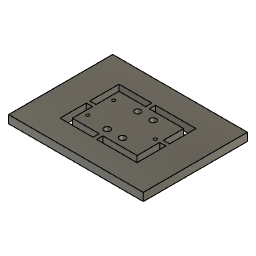
Usinage v5 (Autodesk Fusion 360 design; units mm, degrees)
Autodesk Fusion 360 part; units mm, degrees
sketch "Esquisse1" plane through (0, 0, 0) normal (0, 0, 1) x (1, 0, 0)
  line L0 (-35, 50) -> (75, 50)
  line L1 (75, 50) -> (75, -35)
  line L2 (75, -35) -> (-35, -35)
  line L3 (-35, -35) -> (-35, 50)
  circle A0 centre (28.055, -5) radius 2.5
  circle A1 centre (-2.15, 18) radius 1.25
  circle A2 centre (15.555, -5) radius 2.5
  circle A3 centre (-2.15, -3) radius 1.25
  circle A4 centre (15.555, 20) radius 2.5
  circle A5 centre (42.25, 7.5) radius 1.25
  circle A6 centre (28.055, 20) radius 2.5
  line L4 (-11.4, 4.8329) -> (-6.4, 4.8329)
  line L5 (-11.4, 7.8329) -> (-6.4, 7.8329)
  line L6 (15.3682, 31.55) -> (15.3682, 26.55)
  line L7 (18.3682, 31.55) -> (18.3682, 26.55)
  line L8 (46.4, 10) -> (51.4, 10)
  line L9 (46.4, 7) -> (51.4, 7)
  line L10 (15.555, -11.55) -> (15.555, -16.55)
  line L11 (18.555, -11.55) -> (18.555, -16.55)
  line L12 (-11.4, 31.55) -> (15.3682, 31.55)
  line L13 (18.3682, 31.55) -> (51.4, 31.55)
  line L14 (46.4, 26.55) -> (18.3682, 26.55)
  line L15 (15.3682, 26.55) -> (-6.4, 26.55)
  line L16 (51.4, 31.55) -> (51.4, 10)
  line L17 (51.4, 7) -> (51.4, -16.55)
  line L18 (46.4, -11.55) -> (46.4, 7)
  line L19 (46.4, 10) -> (46.4, 26.55)
  line L20 (-6.4, -11.55) -> (15.555, -11.55)
  line L21 (18.555, -11.55) -> (46.4, -11.55)
  line L22 (51.4, -16.55) -> (18.555, -16.55)
  line L23 (15.555, -16.55) -> (-11.4, -16.55)
  line L24 (-11.4, -16.55) -> (-11.4, 4.8329)
  line L25 (-11.4, 7.8329) -> (-11.4, 31.55)
  line L26 (-6.4, 26.55) -> (-6.4, 7.8329)
  line L27 (-6.4, 4.8329) -> (-6.4, -11.55)
  point P0 (20, 10)
  dimension "d1" = 110
  dimension "d2" = 85
  dimension "d3" = 2.5
  dimension "d4" = 2.5
  dimension "d5" = 5
  dimension "d6" = 5
  dimension "d7" = 5
  dimension "d8" = 5
  dimension "d9" = 2.5
  dimension "d10" = 38.1
  dimension "d11" = 52.8
  dimension "d12" = 6.55
  dimension "d13" = 6.55
  dimension "d14" = 8.55
  dimension "d15" = 8.55
  dimension "d16" = 6.55
  dimension "d17" = 6.55
  dimension "d18" = 19.05
  dimension "d19" = 4.15
  dimension "d20" = 18.345
  dimension "d21" = 30.845
  dimension "d22" = 4.25
  dimension "d23" = 4.25
  dimension "d24" = 21.955
  dimension "d25" = 18.345
  dimension "d26" = 23.45
  dimension "d27" = 38.1
  dimension "d28" = 52.8
  dimension "d30" = 28.6
  dimension "d35" = 5
  dimension "d36" = 5
  dimension "d37" = 5
  dimension "d38" = 5
  dimension "d39" = 3
  dimension "d40" = 3
  dimension "d41" = 3
  dimension "d42" = 3
  constraint horizontal L0
  constraint vertical L1
  constraint horizontal L2
  constraint vertical L3
  constraint parallel L3 L26
  constraint horizontal L12
  constraint vertical L16
  constraint horizontal L22
  constraint vertical L24
  constraint coincident L4.end L26
  constraint perpendicular L4 L26
  constraint coincident L5.start L24
  constraint perpendicular L5 L26
  constraint coincident L6.end L14
  constraint perpendicular L6 L14
  constraint coincident L7.start L12
  constraint perpendicular L7 L14
  constraint coincident L8.start L18
  constraint perpendicular L8 L16
  constraint coincident L9.end L16
  constraint perpendicular L9 L16
  constraint coincident L10.end L22
  constraint perpendicular L10 L22
  constraint coincident L11.start L20
  constraint perpendicular L11 L22
  constraint collinear L12 L13
  constraint collinear L14 L15
  constraint collinear L16 L17
  constraint collinear L18 L19
  constraint collinear L20 L21
  constraint collinear L22 L23
  constraint collinear L24 L25
  constraint collinear L26 L27
  measures "d1" distance of L1 L3
  measures "d2" distance of L0 L2
  measures "d3" diameter of A1
  measures "d4" diameter of A3
  measures "d5" diameter of A4
  measures "d6" diameter of A6
  measures "d7" diameter of A2
  measures "d8" diameter of A0
  measures "d9" diameter of A5
  measures "d10" distance of L15.end L20.start
  measures "d11" distance of L15.end L14.start
  measures "d12" distance of A6.centre L14
  measures "d13" distance of A4.centre L14
  measures "d14" distance of A1.centre L14
  measures "d15" distance of A3.centre L20
  measures "d16" distance of A2.centre L20
  measures "d17" distance of A0.centre L20
  measures "d18" distance of A5.centre L20
  measures "d19" distance of A5.centre L18
  measures "d20" distance of A6.centre L18
  measures "d21" distance of A4.centre L18
  measures "d22" distance of A1.centre L26
  measures "d23" distance of A3.centre L26
  measures "d24" distance of A2.centre L26
  measures "d25" distance of A0.centre L18
  measures "d26" distance of L0 L14
  measures "d27" distance of L18.start L14.start
  measures "d28" distance of L20.start L18.start
  measures "d30" distance of L3 L26
  measures "d35" distance of L24 L26
  measures "d36" distance of L12 L14
  measures "d37" distance of L20 L22
  measures "d38" distance of L16 L18
  measures "d39" distance of L4 L5
  measures "d40" distance of L10 L11
  measures "d41" distance of L8 L9
  measures "d42" distance of L6 L7
extrude "Extrusion3" add sketch "Esquisse1" along normal blind 6.5 contours L0 L1 L2 L3 | A1 | A3 | A5
sketch "Esquisse3" plane through (0, 0, 6.5) normal (0, 0, 1) x (-1, 0, 0)
  circle A0 centre (-15.555, -20) radius 2.5
  circle A1 centre (-28.055, -20) radius 2.5
  line L0 (11.4, -4.8329) -> (6.4, -4.8329)
  line L1 (6.4, -4.8329) -> (6.4, 11.55)
  line L2 (6.4, 11.55) -> (-15.555, 11.55)
  line L3 (-15.555, 11.55) -> (-15.555, 16.55)
  line L4 (-15.555, 16.55) -> (11.4, 16.55)
  line L5 (11.4, 16.55) -> (11.4, -4.8329)
  line L6 (-18.3682, -26.55) -> (-18.3682, -31.55)
  line L7 (-18.3682, -31.55) -> (-51.4, -31.55)
  line L8 (-51.4, -31.55) -> (-51.4, -10)
  line L9 (-51.4, -10) -> (-46.4, -10)
  line L10 (-46.4, -10) -> (-46.4, -26.55)
  line L11 (-46.4, -26.55) -> (-18.3682, -26.55)
  circle A2 centre (-28.055, 5) radius 2.5
  line L12 (-18.555, 16.55) -> (-18.555, 11.55)
  line L13 (-18.555, 11.55) -> (-46.4, 11.55)
  line L14 (-46.4, 11.55) -> (-46.4, -7)
  line L15 (-46.4, -7) -> (-51.4, -7)
  line L16 (-51.4, -7) -> (-51.4, 16.55)
  line L17 (-51.4, 16.55) -> (-18.555, 16.55)
  line L18 (6.4, -7.8329) -> (11.4, -7.8329)
  line L19 (11.4, -7.8329) -> (11.4, -31.55)
  line L20 (11.4, -31.55) -> (-15.3682, -31.55)
  line L21 (-15.3682, -31.55) -> (-15.3682, -26.55)
  line L22 (-15.3682, -26.55) -> (6.4, -26.55)
  line L23 (6.4, -26.55) -> (6.4, -7.8329)
  circle A3 centre (-15.555, 5) radius 2.5
  line L24 (35, 35) -> (-75, 35)
  line L25 (-75, 35) -> (-75, -50)
  line L26 (-75, -50) -> (35, -50)
  line L27 (35, -50) -> (35, 35)
  line L28 (6.4, 35) -> (6.4, -50) construction
  constraint coincident L24 L28.start
  constraint coincident L26 L28.end
  constraint perpendicular L26 L28
extrude "Extrusion4" cut sketch "Esquisse1" along normal blind 6.5 contours A1 | A3 | A5
